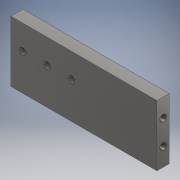
# Autodesk Inventor part: MotorFixer
Saved by Autodesk Inventor 2017 (Build 210142000, 142)
## iProperties
Created: 2016-12-12
Part Number: MotorFixer
Material: Steel, Carbon
Document SubType Name: Modeling
Designer: umr
Density: 7.85 g/cm^3
Appearance: Semi-Polished
Author: umr
Autodesk Inventor part; units mm, degrees
ref_plane "YZ Plane" through (0, 0, 0) normal (1, 0, 0) x (0, 1, 0)
ref_plane "XZ Plane" through (0, 0, 0) normal (0, 1, 0) x (-1, 0, 0)
ref_plane "XY Plane" through (0, 0, 0) normal (0, 0, 1) x (1, 0, 0)
sketch "Sketch1" plane through (0, 0, 0) normal (0, 1, 0) x (-1, 0, 0)
  line L0 (0, 0) -> (120, 0)
  line L1 (120, 0) -> (120, -50)
  line L2 (120, -50) -> (0, -50)
  line L3 (0, -50) -> (0, 0)
  dimension "d0" = 120
  dimension "d1" = 50
  constraints: 8 end point, 2 parallel, 1 horizontal, 1 perpendicular
  measures "d0" distance of L1.end L2.end
  measures "d1" distance of L0.end L1.end
extrude "Extrusion1" add sketch "Sketch1" along normal blind 10
sketch "Sketch2" plane through (0, 10, 0) normal (0, 1, 0) x (1, 0, 0)
  line L0 (-120, 50) -> (-120, 0) projected
  line L1 (-120, 0) -> (0, 0) projected
  circle A0 centre (-110, 20) radius 2.75
  circle A1 centre (-90, 20) radius 2.75
  circle A2 centre (-70, 20) radius 2.75
  dimension "d4" = 5.5
  dimension "d5" = 20
  dimension "d6" = 10
  dimension "d9" = 20
  constraints: 3 centre point, 1 horizontal, 4 other
  measures "d4" diameter of A0
  measures "d5" distance from line of L1 A0.centre
  measures "d6" distance from line of L0 A0.centre
  measures "d9" distance of A0.centre A1.centre
extrude "Extrusion2" cut sketch "Sketch2" against normal blind 10
sketch "Sketch3" plane through (0, 0, 0) normal (1, 0, 0) x (0, 0, -1)
  line L0 (0, 10) -> (50, 10) projected
  line L1 (0, 0) -> (0, 10) projected
  circle A0 centre (15, 5) radius 2.75
  circle A1 centre (35, 5) radius 2.75
  dimension "d16" = 5.5
  dimension "d17" = 50
  dimension "d18" = 10
  dimension "d19" = 5
  dimension "d20" = 15
  dimension "d23" = 20
  constraints: 2 centre point, 1 horizontal, 2 other
  measures "d16" diameter of A0
  measures "d17" distance of L0.start L0.end
  measures "d18" distance of L1.start L0.start
  measures "d19" distance from line of L0 A0.centre
  measures "d20" distance from line of L1 A0.centre
  measures "d23" distance of A0.centre A1.centre
extrude "Extrusion3" cut sketch "Sketch3" against normal blind 8
equation "\"d19\" = 0.5 * d18"
equation "\"d20\" = -0.5 * d23 + 0.5 * d17"
body "Solid1"
